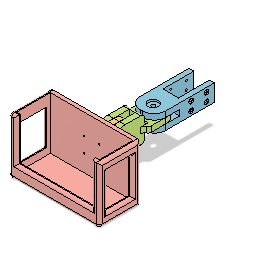
MultimeterHolder (Autodesk Fusion 360 design; units mm, degrees)
part number: MultimeterHolder
Autodesk Fusion 360 part; units mm, degrees
sketch "Sketch1" plane through (0, 0, 0) normal (0, 1, 0) x (1, 0, 0) in component "Holder"
  line L0 (0, 0) -> (96, 0)
  line L1 (96, 0) -> (96, -44)
  line L2 (96, -44) -> (0, -44)
  line L3 (0, -44) -> (0, 0)
  dimension "d4" = 96
  dimension "d5" = 44
  constraint horizontal L0
  constraint vertical L1
  constraint horizontal L2
  constraint vertical L3
  constraint coincident L0.start L3.end
  measures "d4" distance of L0.start L0.end
  measures "d5" distance of L0.start L2.end
extrude "Extrude1" add sketch "Sketch1" along normal blind 60 makes body 1 in component "Holder"
shell "Shell1" thickness 4 removed faces 1 at (32, 60, 14.6667) on bodies 1 in component "Holder"
sketch "Sketch2" plane through (0, 60, 0) normal (0, 1, 0) x (-1, 0, 0) in component "Holder"
  line L0 (-4, 40) -> (-4, 4)
  line L1 (-4, 4) -> (-92, 4)
  line L2 (-92, 4) -> (-92, 40)
  line L3 (-92, 40) -> (-4, 40)
  line L4 (0, 44) -> (-96, 44)
  line L5 (-96, 44) -> (-96, 0)
  line L6 (-96, 0) -> (0, 0)
  line L7 (0, 0) -> (0, 44)
  line L8 (0, 44) -> (-8, 44) construction
  line L9 (-96, 44) -> (-88, 44) construction
  line L10 (-8, 44) -> (-88, 44)
  line L11 (-88, 44) -> (-88, 40)
  line L12 (-88, 40) -> (-8, 40)
  line L13 (-8, 40) -> (-8, 44)
  dimension "d10" = 8
  dimension "d11" = 8
  dimension "d12" = 4
  constraint coincident L4.start L7.end
  constraint perpendicular L7 L8
  constraint coincident L4.end L5.start
  constraint perpendicular L5 L9
  constraint perpendicular L10 L11
  constraint parallel L10 L12
  constraint parallel L11 L13
  measures "d10" distance of L4.start L8.end
  measures "d11" distance of L4.end L9.end
  measures "d12" distance of L8.end L12.end
extrude "Extrude2" cut sketch "Sketch2" against normal blind 45 contours L3 L4 L10 L11 L12 L13 bodies 1 in component "Holder"
sketch "Sketch1 (2)" plane through (0, 0, 0) normal (0, 0, -1) x (-1, 0, 0) in component "Binding1"
  line L0 (-96, 0) -> (0, 0)
  line L1 (0, 0) -> (0, 60)
  line L2 (0, 60) -> (-96, 60)
  line L3 (-96, 60) -> (-96, 0)
  line L4 (-96, 60) -> (0, 0) construction
  line L5 (-34.5, 16.5) -> (-61.5, 16.5)
  line L6 (-61.5, 16.5) -> (-61.5, 43.5)
  line L7 (-61.5, 43.5) -> (-34.5, 43.5)
  line L8 (-34.5, 43.5) -> (-34.5, 16.5)
  line L9 (-34.5, 16.5) -> (-61.5, 43.5) construction
  line L10 (-61.5, 16.5) -> (-34.5, 43.5) construction
  point P0 (-48, 30)
  dimension "d15" = 27
  dimension "d16" = 27
  dimension "d114" = 0
  dimension "d115" = 0
  dimension "d116" = 0
  dimension "d117" = 0
  constraint coincident L2.end L3.start
  constraint coincident L0.end L1.start
  constraint perpendicular L5 L6
  constraint parallel L5 L7
  constraint parallel L6 L8
  constraint horizontal L5
  constraint coincident L9 P0
  constraint coincident L10 P0
  constraint midpoint L4 P0
  measures "d15" distance of L6.end L7.end
  measures "d16" distance of L5.end L6.end
extrude "Extrude1'" add sketch "Sketch1 (2)" along normal blind 4 separate body contours L5 L6 L7 L8 makes body 2 in component "Binding1"
sketch "Sketch3" plane through (0, 0, -4) normal (0, 0, -1) x (-1, 0, 0) in component "Binding1"
  line L0 (-34.5, 43.5) -> (-61.5, 43.5)
  line L1 (-61.5, 43.5) -> (-61.5, 16.5)
  line L2 (-61.5, 16.5) -> (-34.5, 16.5)
  line L3 (-34.5, 16.5) -> (-34.5, 43.5)
  line L4 (-34.5, 27) -> (-61.5, 27)
  line L5 (-61.5, 27) -> (-61.5, 33)
  line L6 (-61.5, 33) -> (-34.5, 33)
  line L7 (-34.5, 33) -> (-34.5, 27)
  line L8 (-34.5, 27) -> (-61.5, 33) construction
  line L9 (-61.5, 27) -> (-34.5, 33) construction
  point P0 (-48, 30)
  point P1 (-48, 30)
  dimension "d21" = 27
  dimension "d22" = 6
  constraint perpendicular L4 L5
  constraint parallel L4 L6
  constraint parallel L5 L7
  constraint horizontal L4
  constraint coincident L8 P1
  constraint coincident L9 P1
  constraint coincident P1 P0
  measures "d21" distance of L5.end L6.end
  measures "d22" distance of L4.end L5.end
extrude "Extrude2'" add sketch "Sketch3" along normal blind 29.2 separate body contours L1 L3 L4 L5 L6 L7 makes body 3 in component "Binding1"
fillet "Fillet1" radius 12.6 2 edges at (61.5, 30, -33.2) (34.5, 30, -33.2) on bodies 3 in component "Binding1"
combine "Combine1" operation add target body 2 tool bodies 3 in component "Binding1"
fillet "Fillet3" radius 4 2 edges at (48, 33, -4) (48, 27, -4) on bodies 2 in component "Binding1"
fillet "Fillet4" radius 4 2 edges at (48, 16.5, -4) (48, 43.5, -4) on bodies 2 in component "Binding1"
sketch "Sketch3 (2)" plane through (0, 0, 0) normal (-1, 0, 0) x (0, 0, 1) in component "Holder"
  line L0 (0, 0) -> (44, 0)
  line L1 (44, 0) -> (44, 60)
  line L2 (44, 60) -> (0, 60)
  line L3 (0, 60) -> (0, 0)
  line L4 (0, 60) -> (44, 0) construction
  line L5 (35.5, 11.25) -> (8.5, 11.25)
  line L6 (8.5, 11.25) -> (8.5, 48.75)
  line L7 (8.5, 48.75) -> (35.5, 48.75)
  line L8 (35.5, 48.75) -> (35.5, 11.25)
  line L9 (35.5, 11.25) -> (8.5, 48.75) construction
  line L10 (8.5, 11.25) -> (35.5, 48.75) construction
  point P0 (22, 30)
  dimension "d70" = 27
  dimension "d71" = 37.5
  constraint coincident L2.end L3.start
  constraint coincident L0.end L1.start
  constraint perpendicular L5 L6
  constraint parallel L5 L7
  constraint parallel L6 L8
  constraint horizontal L5
  constraint coincident L9 P0
  constraint coincident L10 P0
  constraint midpoint L4 P0
  measures "d70" distance of L6.end L7.end
  measures "d71" distance of L5.end L6.end
extrude "Extrude3" cut sketch "Sketch3 (2)" against normal up to surface (96 mm away) contours L5 L6 L7 L8 bodies 1 in component "Holder"
fillet "Fillet1'" radius 3 21 edges at (0, 30, 44) (0, 30, 0) (96, 30, 44) (96, 30, 0) (0, 11.25, 22) (0, 48.75, 22) (0, 30, 8.5) (0, 30, 35.5) (96, 11.25, 22) (96, 48.75, 22) (96, 30, 8.5) (96, 30, 35.5) (96, 60, 22) (96, 0, 22) (0, 0, 22) (0, 60, 22) (4, 60, 44) (8, 37.5, 44) (48, 15, 44) (88, 37.5, 44) (48, 0, 44) on bodies 1 in component "Holder"
sketch "Sketch6" plane through (0, 0, 0) normal (0, 0, -1) x (1, 0, 0) in component "Binding1"
  line L0 (39.9, -21.9) -> (56.1, -21.9) construction
  line L1 (56.1, -21.9) -> (56.1, -38.1) construction
  line L2 (56.1, -38.1) -> (39.9, -38.1) construction
  line L3 (39.9, -38.1) -> (39.9, -21.9) construction
  line L4 (39.9, -21.9) -> (56.1, -38.1) construction
  line L5 (56.1, -21.9) -> (39.9, -38.1) construction
  circle A0 centre (56.1, -38.1) radius 0.75
  circle A1 centre (39.9, -38.1) radius 0.75
  circle A2 centre (56.1, -21.9) radius 0.75
  circle A3 centre (39.9, -21.9) radius 0.75
  point P0 (48, -30)
  point P1 (48, -30)
  dimension "d98" = 16.2
  dimension "d99" = 16.2
  dimension "d100" = 1.5
  dimension "d101" = 1.5
  dimension "d102" = 1.5
  dimension "d103" = 1.5
  constraint perpendicular L0 L1
  constraint parallel L0 L2
  constraint parallel L1 L3
  constraint horizontal L0
  constraint coincident L4 P1
  constraint coincident L5 P1
  constraint coincident P0 P1
  constraint coincident L1.end L2.start
  constraint coincident L2.end L3.start
  constraint coincident L0.end L1.start
  constraint coincident L0.start L3.end
  measures "d98" distance of L1.end L2.end
  measures "d99" distance of L0.end L1.end
  measures "d100" diameter of A0
  measures "d101" diameter of A1
  measures "d102" diameter of A2
  measures "d103" diameter of A3
sketch "Sketch7" plane through (0, 33, 0) normal (0, 1, 0) x (-1, 0, 0) in component "Binding1"
  line L0 (-34.5, -8) -> (-61.5, -8)
  line L1 (-61.5, -8) -> (-61.5, -20.6)
  arc A0 (-61.5, -20.6) -> (-48.9, -33.2) centre (-48.9, -20.6) ccw
  line L2 (-48.9, -33.2) -> (-47.1, -33.2)
  arc A1 (-47.1, -33.2) -> (-34.5, -20.6) centre (-47.1, -20.6) ccw
  line L3 (-34.5, -20.6) -> (-34.5, -8)
  line L4 (-48, -33.2) -> (-48, -8) construction
  circle A2 centre (-48, -20.6) radius 2
  dimension "d106" = 4
  constraint midpoint L2 L4.start
  constraint midpoint L0 L4.end
  constraint midpoint L4 A2.centre
  measures "d106" diameter of A2
extrude "Extrude6" cut sketch "Sketch7" against normal up to surface (6 mm away) contours A2 bodies 2 in component "Binding1"
extrude "Extrude5" cut sketch "Sketch1 (2)" sketch "Sketch6" along normal up to surface of sketch 2 end surface through (0, 0, -4) normal (0, 0, -1) offset 0 bodies 2 in component "Binding1"
ref_plane "WorkPlane2" through (48, 33, -8) normal (0, 0, 1) x (-1, 0, 0) in component "Binding1"
split "Split1" by plane through (48, 33, -8) normal (0, 0, 1) bodies 2 makes body 4 at (50.5167, 27.47, 0) in component "Binding1"
ref_plane "WorkPlane3" through (48, 30, -18.6) normal (0, 1, 0) x (1, 0, 0) in component "Binding1"
copy_body "CopyPasteBodies2" bodies 2 body 2 seen with x (1, 0, 0) y (0, 1, 0) z (0, 0, 1) at (-9.6799, -15.3495, -36.2718) makes body 5 in component "Binding2"
move_body "Move5" bodies 5 to x (-1, 0, 0) y (0, 1, 0) z (0, 0, -1) at (46.1401, 6, -147.3437) in component "Binding2"
move_face "OffsetFaces1" offset 4 1 faces at (3.3201, 21.6505, -103.0718) on bodies 5 in component "Binding2"
copy_body "CopyPasteBodies3" bodies 5 makes body 6 in component "Binding2"
sketch "Sketch6 (2)" plane through (0, 23.6505, 0) normal (0, 1, 0) x (-1, 0, 0) in component "Binding2"
  circle A0 centre (-7.8201, -90.4718) radius 2
  line L0 (-21.3201, -107.0718) -> (5.6799, -107.0718)
  line L1 (5.6799, -107.0718) -> (5.6799, -90.4718)
  arc A1 (5.6799, -90.4718) -> (-6.9201, -77.8718) centre (-6.9201, -90.4718) ccw
  line L2 (-6.9201, -77.8718) -> (-8.7201, -77.8718)
  arc A2 (-8.7201, -77.8718) -> (-21.3201, -90.4718) centre (-8.7201, -90.4718) ccw
  line L3 (-21.3201, -90.4718) -> (-21.3201, -107.0718)
  circle A3 centre (-7.8201, -90.4718) radius 5.5
  dimension "d188" = 11
  constraint concentric A0 A3
  measures "d188" diameter of A3
extrude "Extrude3'" cut sketch "Sketch6 (2)" against normal blind 2 contours A3 bodies 6 5 in component "Binding2"
move_body "Move6" bodies 6 to x (1, 0, 0) y (0, 1, 0) z (0, 0, 1) at (0, -12, 0) in component "Binding2"
sketch "Sketch7 (2)" plane through (0, 0, -107.0718) normal (0, 0, -1) x (-1, 0, 0) in component "Binding2"
  line L0 (5.6799, 5.6505) -> (5.6799, 11.6505)
  line L1 (5.6799, 11.6505) -> (-21.3201, 11.6505)
  line L2 (-21.3201, 11.6505) -> (-21.3201, 5.6505)
  line L3 (-21.3201, 5.6505) -> (5.6799, 5.6505)
  line L4 (-21.3201, 11.6505) -> (5.6799, 5.6505) construction
  point P0 (-7.8201, 8.6505)
  constraint coincident L1.end L2.start
  constraint coincident L0.start L3.end
  constraint midpoint L4 P0
move_body "Move11" bodies 6 to x (-1, 0, 0) y (0, -1, 0) z (0, 0, 1) at (15.7374, 17.0381, 0) in component "Binding2"
sketch "Sketch2 (2)" plane through (0, 0, -107.0718) normal (0, 0, -1) x (-1, 0, 0) in component "Binding2"
  line L0 (5.6799, 17.6505) -> (5.6799, 23.6505)
  line L1 (5.6799, 23.6505) -> (-21.3201, 23.6505)
  line L2 (-21.3201, 23.6505) -> (-21.3201, 17.6505)
  line L3 (-21.3201, 17.6505) -> (5.6799, 17.6505)
extrude "Extrude1''" add sketch "Sketch2 (2)" along normal blind 4 separate body makes body 7 in component "Binding2"
sketch "Sketch3 (3)" plane through (0, 17.6505, 0) normal (0, -1, 0) x (1, 0, 0) in component "Binding2"
  line L0 (21.3201, -107.0718) -> (-5.6799, -107.0718)
  line L1 (-5.6799, -107.0718) -> (-5.6799, -111.0718)
  line L2 (-5.6799, -111.0718) -> (21.3201, -111.0718)
  line L3 (21.3201, -111.0718) -> (21.3201, -107.0718)
extrude "Extrude2''" add sketch "Sketch3 (3)" along normal up to surface (12.2629 mm away) separate body makes body 8 in component "Binding2"
combine "Combine1'" operation add target body 7 tool bodies 8 in component "Binding2"
copy_body "CopyPasteBodies4" bodies 5 makes body 9 in component "Binding2"
move_body "Move8" bodies 9 to x (-1, 0, 0) y (0, 1, 0) z (0, 0, -1) at (15.6401, 0, -180.9437) in component "Binding2"
move_body "Move9" bodies 9 to x (0, 1, 0) y (-1, 0, 0) z (0, 0, 1) at (17.9706, 29.3304, 0) in component "Binding2"
sketch "Sketch4" plane through (0, 0, -111.0718) normal (0, 0, -1) x (-1, 0, 0) in component "Binding2"
  line L0 (5.6799, 5.3876) -> (5.6799, 23.6505)
  line L1 (5.6799, 23.6505) -> (-21.3201, 23.6505)
  line L2 (-21.3201, 23.6505) -> (-21.3201, 5.3876)
  line L3 (-21.3201, 5.3876) -> (5.6799, 5.3876)
  line L4 (-7.8201, 23.6505) -> (-7.8201, 5.3876) construction
  line L5 (-4.8201, 4.1036) -> (-10.8201, 4.1036)
  line L6 (-10.8201, 4.1036) -> (-10.8201, 24.9345)
  line L7 (-10.8201, 24.9345) -> (-4.8201, 24.9345)
  line L8 (-4.8201, 24.9345) -> (-4.8201, 4.1036)
  line L9 (-4.8201, 4.1036) -> (-10.8201, 24.9345) construction
  line L10 (-10.8201, 4.1036) -> (-4.8201, 24.9345) construction
  point P0 (-7.8201, 14.5191)
  dimension "d160" = 6
  constraint midpoint L1 L4.start
  constraint midpoint L3 L4.end
  constraint perpendicular L5 L6
  constraint parallel L5 L7
  constraint parallel L6 L8
  constraint horizontal L5
  constraint coincident L9 P0
  constraint coincident L10 P0
  constraint midpoint L4 P0
  measures "d160" distance of L6.end L7.end
sketch "Sketch5" plane through (0.3201, 0, 0) normal (1, 0, 0) x (0, 0, -1) in component "Binding2"
  circle A0 centre (90.4718, 37.1505) radius 2
  line L0 (73.8718, 50.6505) -> (73.8718, 23.6505)
  line L1 (73.8718, 23.6505) -> (90.4718, 23.6505)
  arc A1 (90.4718, 23.6505) -> (103.0718, 36.2505) centre (90.4718, 36.2505) ccw
  line L2 (103.0718, 36.2505) -> (103.0718, 38.0505)
  arc A2 (103.0718, 38.0505) -> (90.4718, 50.6505) centre (90.4718, 38.0505) ccw
  line L3 (90.4718, 50.6505) -> (73.8718, 50.6505)
  line L4 (73.8718, 37.1505) -> (103.0718, 37.1505) construction
  constraint midpoint L0 L4.start
  constraint midpoint L2 L4.end
move_body "Move10" bodies 9 to x (1, 0, 0) y (0, 1, 0) z (0, 0, 1) at (10.5, -22.6315, -37.2) in component "Binding2"
move_body "Move12" bodies 9 to x (1, 0, 0) y (0, 1, 0) z (0, 0, 1) at (0, 0, -2) in component "Binding2"
move_face "OffsetFaces4" offset 2 1 faces at (6.8201, 10.0191, -113.0718) on bodies 9 in component "Binding2"
move_face "OffsetFaces3" offset 2 1 faces at (6.8201, 10.2951, -128.5848) on bodies 9 in component "Binding2"
combine "Combine3" operation add target body 9 tool bodies 7 6 5 in component "Binding2"
fillet "Fillet2" radius 4 6 edges at (7.8201, 23.6505, -111.0718) (7.8201, 28.0191, -111.0718) (4.8201, 14.5191, -111.0718) (10.8201, 14.5191, -111.0718) (7.8201, 5.3876, -111.0718) (7.8201, 1.0191, -111.0718) on bodies 9 in component "Binding2"
fillet "Fillet2" radius 4 2 edges at (21.3201, 14.5191, -111.0718) (-5.6799, 14.5191, -111.0718) on bodies 9 in component "Binding2"
move_face "OffsetFaces1'" offset 2 1 faces at (43.5, 31, -8) on bodies 2 in component "Binding1"
move_body "Move1" bodies 2 to x (1, 0, 0) y (0, 1, 0) z (0, 0, 1) at (0, 0, -2) in component "Binding1"
copy_body "CopyPasteBodies1" bodies 2 body 2 seen with x (0, -1, 0) y (1, 0, 0) z (0, 0, 1) at (18, 78, 0) makes body 10 in component "Binding3"
move_body "Move1'" bodies 10 to x (0, 1, 0) y (1, 0, 0) z (0, 0, -1) at (31.25, -31.25, -78.8) in component "Binding3"
copy_body "CopyPasteBodies2'" bodies 10 makes body 11 in component "Binding3"
move_body "Move2" bodies 10 to x (1, 0, 0) y (0, 1, 0) z (0, 0, 1) at (0, 12, 0) in component "Binding3"
ref_plane "WorkPlane1" through (61.25, 22.75, -57.2) normal (0, -1, 0) x (1, 0, 0) in component "Binding3"
sketch "Sketch2 (3)" plane through (0, 0, -70.8) normal (0, 0, -1) x (-1, 0, 0) in component "Binding3"
  line L0 (-47.75, 25.75) -> (-47.75, 31.75)
  line L1 (-47.75, 31.75) -> (-74.75, 31.75)
  line L2 (-74.75, 31.75) -> (-74.75, 25.75)
  line L3 (-74.75, 25.75) -> (-47.75, 25.75)
extrude "Extrude2'''" add sketch "Sketch2 (3)" along normal blind 4 separate body makes body 12 in component "Binding3"
sketch "Sketch3 (4)" plane through (0, 25.75, 0) normal (0, -1, 0) x (1, 0, 0) in component "Binding3"
  line L0 (74.75, -70.8) -> (47.75, -70.8)
  line L1 (47.75, -70.8) -> (47.75, -74.8)
  line L2 (47.75, -74.8) -> (74.75, -74.8)
  line L3 (74.75, -74.8) -> (74.75, -70.8)
extrude "Extrude3''" add sketch "Sketch3 (4)" along normal up to surface (12 mm away) bodies 11 10 12 in component "Binding3"
move_face "OffsetFaces1''" offset 33 1 faces at (65.75, 25.75, -74.8) on bodies 11 in component "Binding3"
sketch "Sketch4 (2)" plane through (0, 0, -107.8) normal (0, 0, -1) x (-1, 0, 0) in component "Binding3"
  line L0 (-74.75, 13.75) -> (-47.75, 13.75)
  line L1 (-47.75, 13.75) -> (-47.75, 31.75)
  line L2 (-47.75, 31.75) -> (-74.75, 31.75)
  line L3 (-74.75, 31.75) -> (-74.75, 13.75)
  line L4 (-61.25, 31.75) -> (-61.25, 13.75) construction
  line L5 (-53, 13.75) -> (-69.5, 13.75)
  line L6 (-69.5, 13.75) -> (-69.5, 31.75)
  line L7 (-69.5, 31.75) -> (-53, 31.75)
  line L8 (-53, 31.75) -> (-53, 13.75)
  line L9 (-53, 13.75) -> (-69.5, 31.75) construction
  line L10 (-69.5, 13.75) -> (-53, 31.75) construction
  point P0 (-61.25, 22.75)
  dimension "d256" = 16.5
  constraint midpoint L2 L4.start
  constraint midpoint L0 L4.end
  constraint perpendicular L5 L6
  constraint parallel L5 L7
  constraint parallel L6 L8
  constraint horizontal L5
  constraint coincident L0 L5.start
  constraint coincident L9 P0
  constraint coincident L10 P0
  constraint midpoint L4 P0
  measures "d256" distance of L6.end L7.end
extrude "Extrude4" cut sketch "Sketch4 (2)" against normal blind 33 contours L0 L2 L5 L6 L7 L8 bodies 11 in component "Binding3"
sketch "Sketch5 (2)" plane through (0, 31.75, 0) normal (0, 1, 0) x (-1, 0, 0) in component "Binding3"
  line L0 (-69.5, -107.8) -> (-69.5, -74.8)
  line L1 (-69.5, -74.8) -> (-53, -74.8)
  line L2 (-53, -74.8) -> (-53, -107.8)
  line L3 (-53, -107.8) -> (-47.75, -107.8)
  line L4 (-47.75, -107.8) -> (-47.75, -56.2)
  arc A0 (-47.75, -56.2) -> (-60.35, -43.6) centre (-60.35, -56.2) ccw
  line L5 (-60.35, -43.6) -> (-62.15, -43.6)
  arc A1 (-62.15, -43.6) -> (-74.75, -56.2) centre (-62.15, -56.2) ccw
  line L6 (-74.75, -56.2) -> (-74.75, -107.8)
  line L7 (-74.75, -107.8) -> (-69.5, -107.8)
  circle A2 centre (-61.25, -56.2) radius 2
  circle A3 centre (-61.25, -56.2) radius 5.5
  dimension "d259" = 11
  constraint concentric A2 A3
  measures "d259" diameter of A3
extrude "Extrude5'" cut sketch "Sketch5 (2)" against normal blind 2 contours A3 bodies 11 in component "Binding3"
mirror "Mirror1" about plane through (61.25, 22.75, -57.2) normal (0, -1, 0) of 2 faces at (56.9446, 29.75, -56.5726) (55.7773, 31.0833, -56.7476) on bodies 11 in component "Binding3"
sketch "Sketch6 (3)" plane through (53, 0, 0) normal (1, 0, 0) x (0, 0, -1) in component "Binding3"
  line L0 (107.8, 13.75) -> (107.8, 31.75)
  line L1 (107.8, 31.75) -> (74.8, 31.75)
  line L2 (74.8, 31.75) -> (74.8, 13.75)
  line L3 (74.8, 13.75) -> (107.8, 13.75)
  line L4 (91.3, 31.75) -> (91.3, 13.75) construction
  line L5 (74.8, 31.75) -> (91.3, 22.75) construction
  line L6 (107.8, 13.75) -> (91.3, 22.75) construction
  circle A0 centre (83.05, 27.25) radius 1
  circle A1 centre (99.55, 27.25) radius 1
  line L7 (107.8, 22.75) -> (91.3, 22.75) construction
  circle A2 centre (99.55, 18.25) radius 1
  circle A3 centre (83.05, 18.25) radius 1
  dimension "d263" = 2
  constraint midpoint L1 L4.start
  constraint midpoint L3 L4.end
  constraint coincident L1.end L2.start
  constraint midpoint L4 L5.end
  constraint coincident L0.start L3.end
  constraint midpoint L5 A0.centre
  constraint symmetric L4 A0 A1
  constraint midpoint L0 L7.start
  constraint symmetric A0 L7 A3
  constraint symmetric A1 L7 A2
  measures "d263" diameter of A0
extrude "Extrude6'" cut sketch "Sketch6 (3)" along normal up to surface (21.75 mm away) and the other way up to surface (5.25 mm away) contours A0 | A1 | A2 | A3 bodies 11 in component "Binding3"
sketch "Sketch5 (3)" plane through (0, 0, 4) normal (0, 0, 1) x (1, 0, 0) in component "Holder"
  line L0 (4, 4) -> (92, 4)
  line L1 (92, 4) -> (92, 60)
  line L2 (92, 60) -> (4, 60)
  line L3 (4, 60) -> (4, 4)
  circle A0 centre (39.9, 38.1) radius 0.75
  circle A1 centre (56.1, 38.1) radius 0.75
  circle A2 centre (56.1, 21.9) radius 0.75
  circle A3 centre (39.9, 21.9) radius 0.75
extrude "Extrude5''" cut sketch "Sketch5 (3)" against normal up to surface (4 mm away) contours A0 | A1 | A2 | A3 bodies 1 in component "Holder"
sketch "Sketch7 (3)" plane through (74.75, 0, 0) normal (1, 0, 0) x (0, 0, -1) in component "Binding3"
  circle A0 centre (83.05, 18.25) radius 1
  circle A1 centre (99.55, 27.25) radius 1
  circle A2 centre (83.05, 27.25) radius 1
  circle A3 centre (99.55, 18.25) radius 1
  line L0 (70.8, 19.75) -> (56.2, 19.75)
  line L1 (56.2, 19.75) -> (56.2, 13.75)
  line L2 (56.2, 13.75) -> (107.8, 13.75)
  line L3 (107.8, 13.75) -> (107.8, 31.75)
  line L4 (107.8, 31.75) -> (56.2, 31.75)
  line L5 (56.2, 31.75) -> (56.2, 25.75)
  line L6 (56.2, 25.75) -> (70.8, 25.75)
  line L7 (70.8, 25.75) -> (70.8, 19.75)
  circle A4 centre (83.05, 27.25) radius 2.5
  circle A5 centre (99.55, 27.25) radius 2.5
  circle A6 centre (83.05, 18.25) radius 2.5
  circle A7 centre (99.55, 18.25) radius 2.5
  dimension "d270" = 5
  dimension "d271" = 5
  dimension "d272" = 5
  dimension "d273" = 5
  constraint concentric A2 A4
  constraint concentric A1 A5
  constraint concentric A0 A6
  constraint concentric A3 A7
  measures "d270" diameter of A4
  measures "d271" diameter of A5
  measures "d272" diameter of A6
  measures "d273" diameter of A7
extrude "Extrude7" cut sketch "Sketch7 (3)" against normal blind 1 contours A4 | A5 | A6 | A7 bodies 11 in component "Binding3"
ref_plane "WorkPlane2" through (61.25, 22.75, -91.3) normal (1, 0, 0) x (0, 1, 0) in component "Binding3"
mirror "Mirror2" about plane through (61.25, 22.75, -91.3) normal (1, 0, 0) of 8 faces at (73.75, 27.1258, -85.0407) (73.75, 29.0577, -98.7071) (73.75, 19.513, -81.5062) (73.75, 16.4639, -98.6622) (74.4167, 18.0011, -102.0376) (74.0833, 19.7595, -81.0572) (74.4167, 27.0011, -85.5376) (74.0833, 28.857, -101.4651) on bodies 11 in component "Binding3"
component "Holder" placed x (1, 0, 0) y (0, 1, 0) z (0, 0, 1) at (0, 0, 0)
component "Binding1" placed x (0, -1, 0) y (1, 0, 0) z (0, 0, 1) at (18, 78, 0)
component "Binding2" placed x (0, -1, 0) y (1, 0, 0) z (0, 0, 1) at (33.3495, 37.8201, 67.8718)
component "Binding3" placed x (1, 0, 0) y (0, 1, 0) z (0, 0, 1) at (-13.3815, 7.25, -5.6)
equation "width = 88 mm"
equation "depth = 36 mm"
equation "bottomConnectorsDistance = 15 mm"
equation "d4 = width + wallThickness * 2"
equation "d5 = depth + wallThickness * 2"
equation "wallThickness = 4 mm"
equation "d7 = bottomConnectorsDistance * 4"
equation "d9 = wallThickness"
equation "d10 = wallThickness * 2"
equation "d11 = wallThickness * 2"
equation "d12 = wallThickness"
equation "d13 = -bottomConnectorsDistance * 3"
equation "d15 = depth * 0.75"
equation "d16 = depth * 0.75"
equation "d17 = wallThickness"
equation "d21 = depth * 0.75"
equation "d22 = wallThickness * 1.5"
equation "d23 = depth * 0.7 + wallThickness"
equation "d25 = depth * 0.35"
equation "bindingScrewDiam = 4 mm"
equation "furnitureWallThickness = 16.5 mm"
equation "d68 = wallThickness"
equation "d69 = wallThickness"
equation "d70 = depth * 0.75"
equation "d71 = bottomConnectorsDistance * 2.5"
equation "d74 = wallThickness * 0.75"
equation "d98 = depth * 0.45"
equation "d99 = depth * 0.45"
equation "d106 = bindingScrewDiam"
equation "d153 = wallThickness"
equation "d154 = wallThickness"
equation "d160 = wallThickness * 1.5"
equation "d188 = bindingScrewDiam * 2.75"
equation "d195 = wallThickness"
equation "d244 = wallThickness"
equation "d246 = wallThickness * 1.5 * 2"
equation "d251 = wallThickness"
equation "d255 = furnitureWallThickness * 2"
equation "d256 = furnitureWallThickness"
equation "d257 = -furnitureWallThickness * 2"
equation "d259 = bindingScrewDiam * 2.75"
equation "d260 = -wallThickness * 0.5"
